Autodesk Fusion 360 part; units mm, degrees
(part 2 of 4)
sketch "Boceto28" plane through (0, 68, 0) normal (0, 1, 0) x (-1, 0, 0)
  line L0 (-4.7, -42.05) -> (43.7, -42.05)
  line L1 (43.7, -42.05) -> (43.7, -11.65)
  line L2 (43.7, -11.65) -> (-4.7, -11.65)
  line L3 (-4.7, -11.65) -> (-4.7, -42.05)
  line L4 (83, -73) -> (83, 19.3)
  line L5 (-44, -73) -> (83, -73)
  line L6 (-44, 19.3) -> (-44, -73)
  line L7 (83, 19.3) -> (-44, 19.3)
  line L8 (-33, -6.85) -> (72, -6.85)
  line L9 (72, -6.85) -> (72, -46.85)
  line L10 (72, -46.85) -> (-33, -46.85)
  line L11 (-33, -46.85) -> (-33, -6.85)
  line L12 (-33, -6.85) -> (72, -46.85) construction
  line L13 (72, -6.85) -> (-33, -46.85) construction
  point P0 (19.5, -26.85)
  point P1 (19.5, -26.85)
  dimension "d98" = 40
  dimension "d99" = 105
  constraint horizontal L8
  constraint perpendicular L8 L9
  constraint parallel L8 L10
  constraint parallel L9 L11
  constraint coincident L12 P1
  constraint coincident L13 P1
  constraint coincident P1 P0
  measures "d98" distance of L8.end L9.end
  measures "d99" distance of L9.end L10.end
extrude "Extruir27" add sketch "Boceto28" along normal blind 15 separate body contours L4 L5 L6 L7 makes body 3
sketch "Boceto29" plane through (0, 68, 0) normal (0, -1, 0) x (1, 0, 0)
  line L0 (33, -46.85) -> (-72, -46.85)
  line L1 (-72, -46.85) -> (-72, -6.85)
  line L2 (-72, -6.85) -> (33, -6.85)
  line L3 (33, -6.85) -> (33, -46.85)
  line L4 (44, 19.3) -> (-83, 19.3)
  line L5 (-83, 19.3) -> (-83, -73)
  line L6 (-83, -73) -> (44, -73)
  line L7 (44, -73) -> (44, 19.3)
  line L8 (33, -46.85) -> (33, -6.85)
  line L9 (-72, -46.85) -> (33, -46.85)
  line L10 (33, -6.85) -> (-72, -6.85)
  line L11 (-72, -6.85) -> (-72, -46.85)
  line L12 (-72, -6.85) -> (33, -6.85)
  line L13 (33, -6.85) -> (33, -46.85)
  line L14 (33, -46.85) -> (-72, -46.85)
  line L15 (-72, -46.85) -> (-72, -6.85)
  line L16 (30, -43.85) -> (-69, -43.85)
  line L17 (-69, -43.85) -> (-69, -9.85)
  line L18 (-69, -9.85) -> (30, -9.85)
  line L19 (30, -9.85) -> (30, -43.85)
  line L20 (-75, -49.85) -> (-75, -3.85)
  line L21 (-75, -3.85) -> (36, -3.85)
  line L22 (36, -3.85) -> (36, -49.85)
  line L23 (36, -49.85) -> (-75, -49.85)
  dimension "d102" = 3
  dimension "d103" = -3
  constraint horizontal L12
  constraint vertical L13
  constraint horizontal L14
  constraint vertical L15
  constraint coincident L0.start L3.end
  constraint coincident L1.end L2.start
extrude "Extruir28" add sketch "Boceto29" along normal blind 5 contours L0 L1 L2 L3 L8 L9 L10 L11 L12 L13 L14 L15 | L20 L21 L22 L23 bodies 3
sketch "Boceto30" plane through (0, 46, 0) normal (0, 1, 0) x (-1, 0, 0)
  line L0 (-41, -18.85) -> (-37, -18.85)
  line L1 (-37, -18.85) -> (-37, -22.85)
  line L2 (-37, -22.85) -> (-41, -22.85)
  line L3 (-41, -22.85) -> (-41, -30.85)
  line L4 (-41, -30.85) -> (-37, -30.85)
  line L5 (-37, -30.85) -> (-37, -34.85)
  line L6 (-37, -34.85) -> (-41, -34.85)
  line L7 (-41, -34.85) -> (-41, -70)
  line L8 (-41, -70) -> (80, -70)
  line L9 (80, -70) -> (80, -34.85)
  line L10 (80, -34.85) -> (76, -34.85)
  line L11 (76, -34.85) -> (76, -30.85)
  line L12 (76, -30.85) -> (80, -30.85)
  line L13 (80, -30.85) -> (80, -22.85)
  line L14 (80, -22.85) -> (76, -22.85)
  line L15 (76, -22.85) -> (76, -18.85)
  line L16 (76, -18.85) -> (80, -18.85)
  line L17 (80, -18.85) -> (80, 16.3)
  line L18 (80, 16.3) -> (-41, 16.3)
  line L19 (-41, 16.3) -> (-41, -18.85)
  line L20 (30, -11.35) -> (60, -11.35)
  line L21 (60, -11.35) -> (60, -42.35)
  line L22 (60, -42.35) -> (30, -42.35)
  line L23 (30, -42.35) -> (30, -43.35)
  line L24 (30, -43.35) -> (9, -43.35)
  line L25 (9, -43.35) -> (9, -10.35)
  line L26 (9, -10.35) -> (30, -10.35)
  line L27 (30, -10.35) -> (30, -11.35)
  line L28 (80, -70) -> (-41, 16.3)
  line L29 (80, 16.3) -> (-41, -70)
  line L30 (-41, 16.3) -> (-28.7879, 7.59)
  line L31 (-41, -70) -> (-28.7879, -61.29)
  line L32 (80, -70) -> (67.7879, -61.29) construction
  line L33 (80, 16.3) -> (67.7879, 7.59)
  circle A0 centre (67.7879, 7.59) radius 2.5
  circle A1 centre (67.7879, -61.29) radius 2.5
  circle A2 centre (-28.7879, -61.29) radius 2.5
  circle A3 centre (-28.7879, 7.59) radius 2.5
  dimension "d106" = 15
  dimension "d107" = 15
  dimension "d108" = 15
  dimension "d109" = 15
  dimension "d110" = 5
  dimension "d111" = 5
  dimension "d112" = 5
  dimension "d113" = 5
  constraint coincident L18.end L19.start
  constraint parallel L28 L30
  constraint coincident L7.end L8.start
  constraint parallel L29 L31
  constraint coincident L8.end L9.start
  constraint parallel L28 L32
  constraint coincident L17.end L18.start
  constraint parallel L29 L33
  constraint coincident L33.end A0.centre
  constraint coincident L32.end A1.centre
  constraint coincident L31.end A2.centre
  constraint coincident L30.end A3.centre
  measures "d106" distance of L18.end L30.end
  measures "d107" distance of L7.end L31.end
  measures "d108" distance of L8.end L32.end
  measures "d109" distance of L17.end L33.end
  measures "d110" diameter of A0
  measures "d111" diameter of A1
  measures "d112" diameter of A2
  measures "d113" diameter of A3
extrude "Extruir29" add sketch "Boceto30" along normal blind 21.99 contours L28 L30 A3 | L28 L30 A3 | L29 L33 A0 | L29 L33 A0 | L29 L31 A2 | L29 L31 A2 | L28 A1 | L28 A1 bodies 2
sketch "Boceto31" plane through (0, 68, 0) normal (0, -1, 0) x (1, 0, 0)
  line L0 (36, -49.85) -> (-75, -49.85)
  line L1 (-75, -49.85) -> (-75, -3.85)
  line L2 (-75, -3.85) -> (36, -3.85)
  line L3 (36, -3.85) -> (36, -49.85)
  line L4 (44, 19.3) -> (-83, 19.3)
  line L5 (-83, 19.3) -> (-83, -73)
  line L6 (-83, -73) -> (44, -73)
  line L7 (44, -73) -> (44, 19.3)
  circle A0 centre (-67.7879, -61.29) radius 2.5
  circle A1 centre (28.7879, -61.29) radius 2.5
  circle A2 centre (28.7879, 7.59) radius 2.5
  circle A3 centre (-67.7879, 7.59) radius 2.5
  circle A4 centre (28.7879, -61.29) radius 4
  circle A5 centre (-67.7879, -61.29) radius 4
  circle A6 centre (28.7879, -61.29) radius 2.5
  circle A7 centre (28.7879, 7.59) radius 2.5
  circle A8 centre (28.7879, 7.59) radius 2.5
  circle A9 centre (-67.7879, 7.59) radius 2.5
  circle A10 centre (28.7879, 7.59) radius 4
  circle A11 centre (-67.7879, 7.59) radius 4
  point P0 (28.7879, 7.59)
  dimension "d116" = 1.5
  dimension "d117" = 1.5
  dimension "d118" = 5
  dimension "d119" = 5
  dimension "d120" = 5
  dimension "d121" = 1.5
  dimension "d122" = 1.5
  constraint concentric A1 A6
  constraint coincident P0 A2.centre
  constraint concentric A2 A8
  constraint concentric A3 A9
  measures "d118" diameter of A6
  measures "d119" diameter of A8
  measures "d120" diameter of A9
extrude "Extruir30" add sketch "Boceto31" along normal blind 6 contours A4 | A5 | A10 | A11 bodies 3
sketch "Boceto32" plane through (0, 0, 19.3) normal (0, 0, 1) x (1, 0, 0)
  circle A0 centre (-18.2562, 20.244) radius 7.405
  line L0 (44, -4) -> (44, 64.2)
  line L1 (44, 64.2) -> (-83, 64.2)
  line L2 (-83, 64.2) -> (-83, -4)
  line L3 (-83, -4) -> (44, -4)
sketch "Boceto33" plane through (-83, 0, 0) normal (-1, 0, 0) x (0, 0, 1)
  line L0 (19.3, -4) -> (19.3, 64.2)
  line L1 (19.3, 64.2) -> (-73, 64.2)
  line L2 (-73, 64.2) -> (-73, -4)
  line L3 (-73, -4) -> (19.3, -4)
sketch "Boceto34" plane through (0, 0, 19.3) normal (0, 0, 1) x (1, 0, 0)
  line L0 (-34.8461, 5.5811) -> (-70.8461, 5.5811)
  line L1 (-70.8461, 5.5811) -> (-70.8461, 39.5811)
  line L2 (-70.8461, 39.5811) -> (-34.8461, 39.5811)
  line L3 (-34.8461, 39.5811) -> (-34.8461, 5.5811)
  line L4 (-34.8461, 5.5811) -> (-70.8461, 39.5811) construction
  line L5 (-70.8461, 5.5811) -> (-34.8461, 39.5811)
  line L6 (-52.8461, 5.5811) -> (-52.8461, 10.5811) construction
  line L7 (-70.3461, 33.5811) -> (-35.3461, 33.5811)
  line L8 (-35.3461, 33.5811) -> (-35.3461, 10.5811)
  line L9 (-35.3461, 10.5811) -> (-70.3461, 10.5811)
  line L10 (-70.3461, 10.5811) -> (-70.3461, 33.5811)
  line L11 (-70.3461, 33.5811) -> (-70.8461, 33.5811) construction
  line L12 (-70.8461, 5.5811) -> (-67.938, 8.3276)
  line L13 (-34.8461, 5.5811) -> (-37.7542, 8.3276)
  line L14 (-70.8461, 39.5811) -> (-67.938, 36.8346)
  line L15 (-34.8461, 39.5811) -> (-37.7542, 36.8346)
  circle A0 centre (-67.938, 8.3276) radius 1.5
  circle A1 centre (-37.7542, 8.3276) radius 1.5
  circle A2 centre (-67.938, 36.8346) radius 1.5
  circle A3 centre (-37.7542, 36.8346) radius 1.5
  line L16 (-70.3461, 33.5811) -> (-35.3461, 33.5811)
  line L17 (-35.3461, 33.5811) -> (-35.3461, 10.5811)
  line L18 (-35.3461, 10.5811) -> (-70.3461, 10.5811)
  line L19 (-70.3461, 10.5811) -> (-70.3461, 33.5811)
  point P0 (-52.8461, 22.5811)
  point P1 (-52.8461, 22.5811)
  dimension "d125" = 34
  dimension "d126" = 36
  dimension "d127" = 5
  dimension "d128" = 23
  dimension "d129" = 35
  dimension "d130" = 0.5
  dimension "d131" = 4
  dimension "d132" = 4
  dimension "d133" = 4
  dimension "d134" = 4
  dimension "d135" = 3
  dimension "d136" = 3
  dimension "d137" = 3
  dimension "d138" = 3
  constraint horizontal L0
  constraint perpendicular L0 L1
  constraint parallel L0 L2
  constraint parallel L1 L3
  constraint coincident L4 P1
  constraint coincident L5 P1
  constraint coincident P0 P1
  constraint midpoint L0 L6.start
  constraint perpendicular L0 L6
  constraint horizontal L7
  constraint vertical L8
  constraint horizontal L9
  constraint vertical L10
  constraint coincident L6.end L9
  constraint coincident L1 L11.end
  constraint perpendicular L1 L11
  constraint parallel L5 L12
  constraint parallel L4 L13
  constraint parallel L4 L14
  constraint parallel L5 L15
  constraint coincident L12.end A0.centre
  constraint coincident L13.end A1.centre
  constraint coincident L14.end A2.centre
  constraint coincident L15.end A3.centre
  constraint horizontal L16
  constraint vertical L17
  constraint horizontal L18
  constraint vertical L19
  measures "d125" distance of L0.end L1.end
  measures "d126" distance of L1.end L2.end
  measures "d127" distance of L6.start L6.end
  measures "d128" distance of L7.start L9.end
  measures "d129" distance of L7.start L7.end
  measures "d130" distance of L7.start L11.end
  measures "d131" distance of L0.end L12.end
  measures "d132" distance of L0.start L13.end
  measures "d133" distance of L1.end L14.end
  measures "d134" distance of L2.end L15.end
  measures "d135" diameter of A0
  measures "d136" diameter of A1
  measures "d137" diameter of A2
  measures "d138" diameter of A3
extrude "Extruir31" add sketch "Boceto34" against normal blind 9 contours L5 L12 A0 | L5 L12 A0 | L5 L15 A3 | L5 L15 A3 | A1 | A2 bodies 1
extrude "Extruir32" cut sketch "Boceto34" against normal blind 6 contours L5 L7 L9 L10 L16 L18 L19 | L5 L7 L8 L9 L16 L17 L18 bodies 1
sketch "Boceto35" plane through (0, 0, 0) normal (0, 1, 0) x (-1, 0, 0)
  line L0 (46.4591, -65.3063) -> (43.7876, -62.6347)
  line L1 (43.7876, -62.6347) -> (43.7876, -12.7779)
  line L2 (43.7876, -12.7779) -> (46.4591, -10.1063)
  line L3 (46.4591, -10.1063) -> (73.416, -10.1063)
  line L4 (73.416, -10.1063) -> (76.0876, -12.7779)
  line L5 (76.0876, -12.7779) -> (76.0876, -62.6347)
  line L6 (76.0876, -62.6347) -> (73.416, -65.3063)
  line L7 (73.416, -65.3063) -> (46.4591, -65.3063)
  line L8 (-41, 16.3) -> (-41, -70)
  line L9 (-41, -70) -> (80, -70)
  line L10 (80, -70) -> (80, 16.3)
  line L11 (80, 16.3) -> (-41, 16.3)
  line L12 (-38.4075, -60.7714) -> (-38.4075, -28.7305)
  line L13 (-38.4075, -28.7305) -> (19.6738, -28.7305)
  line L14 (19.6738, -28.7305) -> (19.6738, -60.7714)
  line L15 (19.6738, -60.7714) -> (-38.4075, -60.7714)
  line L16 (-21.368, 14.2774) -> (-27.5689, 14.2774)
  line L17 (-24.1184, -1.7226) -> (-24.1184, -0.7226)
  line L18 (-20.1184, -0.7226) -> (-18.6184, -0.7226)
  line L19 (-29.0184, -1.7226) -> (-29.0184, -0.7226)
  line L20 (-19.5184, -10.1726) -> (-22.0184, -10.1726)
  line L21 (-30.8184, 3.6774) -> (-30.8184, 5.0774)
  line L22 (-30.2184, -7.6726) -> (-30.2184, -10.1726)
  line L23 (-20.3184, 15.9774) -> (-21.368, 14.2774)
  line L24 (-32.7184, 12.4274) -> (-32.7184, 14.9274)
  line L25 (-22.1184, -1.7226) -> (-24.1184, -1.7226)
  line L26 (-30.8184, 5.0774) -> (-29.9184, 5.0774)
  line L27 (-29.6184, 9.9774) -> (-29.6184, 8.1774)
  line L28 (-29.6184, 8.1774) -> (-30.8184, 8.1774)
  line L29 (-33.1184, 15.9774) -> (-33.1184, -10.3226)
  line L30 (-30.2184, -10.1726) -> (-32.7184, -10.1726)
  line L31 (-27.5184, -1.7226) -> (-29.0184, -1.7226)
  line L32 (-22.0184, -10.1726) -> (-22.0184, -7.6726)
  line L33 (-29.9184, 5.0774) -> (-29.9184, 3.6774)
  line L34 (-30.8184, 8.1774) -> (-30.8184, 9.9774)
  line L35 (-30.8184, 9.9774) -> (-29.6184, 9.9774)
  line L36 (-18.8184, 3.7774) -> (-19.7184, 3.7774)
  line L37 (-18.6184, -0.7226) -> (-18.6184, -1.7226)
  line L38 (-19.7184, 3.7774) -> (-19.7184, 5.1774)
  line L39 (-22.1184, -0.7226) -> (-22.1184, -1.7226)
  line L40 (-19.7184, 5.1774) -> (-18.8184, 5.1774)
  line L41 (-18.8184, 9.7774) -> (-18.8184, 8.3774)
  line L42 (-18.8184, 8.3774) -> (-19.7184, 8.3774)
  line L43 (-19.7184, 8.3774) -> (-19.7184, 9.7774)
  line L44 (-18.8184, 5.1774) -> (-18.8184, 3.7774)
  line L45 (-19.7184, 9.7774) -> (-18.8184, 9.7774)
  line L46 (-15.8184, -10.3226) -> (-15.8184, 15.9774)
  line L47 (-33.1184, -10.3226) -> (-15.8184, -10.3226)
  line L48 (-30.2184, 14.9274) -> (-30.2184, 12.4274)
  line L49 (-30.2184, 12.4274) -> (-32.7184, 12.4274)
  line L50 (-27.5689, 14.2774) -> (-28.6184, 15.9774)
  line L51 (-29.4184, -7.6726) -> (-26.9184, -7.6726)
  line L52 (-32.7184, 14.9274) -> (-30.2184, 14.9274)
  line L53 (-28.6184, 15.9774) -> (-33.1184, 15.9774)
  line L54 (-16.2184, 14.9274) -> (-16.2184, 12.4274)
  line L55 (-22.0184, -7.6726) -> (-19.5184, -7.6726)
  line L56 (-19.5184, -7.6726) -> (-19.5184, -10.1726)
  line L57 (-18.7184, 12.4274) -> (-18.7184, 14.9274)
  line L58 (-24.1184, -0.7226) -> (-22.1184, -0.7226)
  line L59 (-22.1184, 0.6774) -> (-24.1184, 0.6774)
  line L60 (-24.1184, 1.6774) -> (-22.1184, 1.6774)
  line L61 (-15.8184, 15.9774) -> (-20.3184, 15.9774)
  line L62 (-32.7184, -7.6726) -> (-30.2184, -7.6726)
  line L63 (-26.9184, -7.6726) -> (-26.9184, -10.1726)
  line L64 (-18.7184, 14.9274) -> (-16.2184, 14.9274)
  line L65 (-16.2184, 12.4274) -> (-18.7184, 12.4274)
  line L66 (-32.7184, -10.1726) -> (-32.7184, -7.6726)
  line L67 (-27.5184, -0.7226) -> (-27.5184, -1.7226)
  line L68 (-29.0184, -0.7226) -> (-27.5184, -0.7226)
  line L69 (-24.1184, 0.6774) -> (-24.1184, 1.6774)
  line L70 (-29.9184, 3.6774) -> (-30.8184, 3.6774)
  line L71 (-29.4184, -10.1726) -> (-29.4184, -7.6726)
  line L72 (-26.9184, -10.1726) -> (-29.4184, -10.1726)
  line L73 (-18.6184, -1.7226) -> (-20.1184, -1.7226)
  line L74 (-22.1184, 1.6774) -> (-22.1184, 0.6774)
  line L75 (-20.1184, -1.7226) -> (-20.1184, -0.7226)
  line L76 (-23.4598, -8.7741) -> (-23.4598, -9.0434)
  line L77 (-23.1906, -9.0434) -> (-23.1906, -9.1588)
  spline S0 degree 3 poles (-23.0111, -8.4082) (-23.0132, -8.4184) (-23.0174, -8.4383) (-23.0264, -8.4666) (-23.038, -8.4923) (-23.0513, -8.5159) (-23.0675, -8.5367) (-23.0864, -8.5549) (-23.1077, -8.5709) (-23.1316, -8.584) (-23.1575, -8.5944) (-23.1849, -8.602) (-23.2138, -8.6065) (-23.2334, -8.6071) (-23.2435, -8.6075) knots 0 0 0 0 0.093348 0.18081 0.264145 0.343818 0.421385 0.498357 0.576984 0.657917 0.740639 0.825197 0.91066 1 1 1 1
  line L78 (-32.376, 1.6706) -> (-32.376, 1.2172)
  line L79 (-32.4914, 1.2415) -> (-32.4914, 1.8455)
  line L80 (-23.5752, -9.0434) -> (-23.5752, -8.7741)
  line L81 (-32.4914, 0.4031) -> (-32.2094, 0.4482)
  spline S1 degree 3 poles (-31.8408, 1.2717) (-31.8351, 1.2693) (-31.8237, 1.2643) (-31.8055, 1.2594) (-31.7866, 1.2563) (-31.7737, 1.2559) (-31.7673, 1.2557) knots 0 0 0 0 0.24526 0.491995 0.743436 1 1 1 1
  line L82 (-23.4598, -9.0434) -> (-23.1906, -9.0434)
  line L83 (-24.0111, -7.787) -> (-23.0111, -7.9939)
  spline S2 degree 3 poles (-31.4914, 1.4364) (-31.4918, 1.4223) (-31.4926, 1.3947) (-31.4996, 1.3545) (-31.5109, 1.3162) (-31.5264, 1.2802) (-31.546, 1.2474) (-31.5698, 1.2188) (-31.597, 1.1941) (-31.6278, 1.1748) (-31.6602, 1.1594) (-31.6938, 1.1486) (-31.7278, 1.1416) (-31.7508, 1.1407) (-31.7622, 1.1403) knots 0 0 0 0 0.09377 0.184231 0.27213 0.359606 0.445026 0.526727 0.607566 0.688585 0.76897 0.84681 0.923592 1 1 1 1
  spline S3 degree 3 poles (-25.5624, -8.5812) (-25.5645, -8.5915) (-25.5687, -8.6114) (-25.5777, -8.6397) (-25.5892, -8.6654) (-25.6026, -8.689) (-25.6187, -8.7098) (-25.6377, -8.728) (-25.659, -8.744) (-25.6829, -8.7571) (-25.7088, -8.7675) (-25.7362, -8.7751) (-25.7651, -8.7796) (-25.7847, -8.7802) (-25.7947, -8.7806) knots 0 0 0 0 0.093348 0.18081 0.264145 0.343818 0.421385 0.498357 0.576984 0.657917 0.740639 0.825197 0.91066 1 1 1 1
  spline S4 degree 3 poles (-32.4914, 1.8455) (-32.4772, 1.8421) (-32.4498, 1.8357) (-32.4109, 1.8232) (-32.3756, 1.8088) (-32.3433, 1.7924) (-32.3135, 1.7733) (-32.2846, 1.752) (-32.2566, 1.7277) (-32.2337, 1.7049) (-32.2146, 1.6839) (-32.1981, 1.6646) (-32.179, 1.6422) (-32.158, 1.6165) (-32.1348, 1.5874) (-32.1093, 1.5552) (-32.0817, 1.5195) (-32.0626, 1.4946) (-32.0527, 1.4817) knots 0 0 0 0 0.074725 0.144044 0.209069 0.269783 0.329265 0.390134 0.45341 0.518937 0.555488 0.598884 0.649104 0.705717 0.769214 0.839335 0.916353 1 1 1 1
  spline S5 degree 3 poles (-26.0373, -8.6271) (-26.042, -8.6383) (-26.051, -8.66) (-26.07, -8.6889) (-26.0921, -8.7134) (-26.1176, -8.7334) (-26.1458, -8.749) (-26.1766, -8.7596) (-26.2095, -8.7666) (-26.2322, -8.7673) (-26.2439, -8.7677) knots 0 0 0 0 0.135771 0.263552 0.384992 0.505027 0.624716 0.745551 0.869397 1 1 1 1
  line L84 (-23.4598, -9.428) -> (-23.5752, -9.428)
  line L85 (-32.2094, 0.8701) -> (-32.4914, 1.0225)
  spline S6 degree 3 poles (-31.6068, 1.4326) (-31.607, 1.4387) (-31.6073, 1.4506) (-31.6096, 1.4682) (-31.6131, 1.4853) (-31.6184, 1.5018) (-31.625, 1.5177) (-31.6333, 1.5329) (-31.6429, 1.5476) (-31.654, 1.5618) (-31.6667, 1.5752) (-31.6814, 1.5875) (-31.6979, 1.5989) (-31.7161, 1.6093) (-31.7361, 1.6185) (-31.7578, 1.6269) (-31.7814, 1.6343) (-31.7979, 1.6383) (-31.8063, 1.6403) knots 0 0 0 0 0.058001 0.11384 0.169165 0.223941 0.278457 0.333444 0.389076 0.445762 0.504761 0.564849 0.628439 0.695178 0.764689 0.838477 0.917221 1 1 1 1
  line L86 (-31.4914, 0.5967) -> (-31.4914, 0.459)
  spline S7 degree 3 poles (-25.7947, -8.7806) (-25.8082, -8.7801) (-25.8345, -8.7792) (-25.8727, -8.7721) (-25.9083, -8.7602) (-25.9359, -8.7464) (-25.9566, -8.7331) (-25.971, -8.7216) (-25.9845, -8.709) (-25.9969, -8.695) (-26.0086, -8.68) (-26.0192, -8.6635) (-26.0288, -8.6458) (-26.0345, -8.6334) (-26.0373, -8.6271) knots 0 0 0 0 0.13183 0.257674 0.379204 0.49925 0.559358 0.619481 0.679692 0.740425 0.802498 0.866422 0.932049 1 1 1 1
  spline S8 degree 3 poles (-23.486, -8.454) (-23.4907, -8.4652) (-23.4998, -8.4869) (-23.5187, -8.5158) (-23.5408, -8.5404) (-23.5663, -8.5603) (-23.5945, -8.5759) (-23.6253, -8.5866) (-23.6582, -8.5935) (-23.6809, -8.5943) (-23.6926, -8.5947) knots 0 0 0 0 0.135771 0.263552 0.384992 0.505027 0.624716 0.745551 0.869397 1 1 1 1
  spline S9 degree 3 poles (-31.7891, 1.7557) (-31.7778, 1.754) (-31.7558, 1.7506) (-31.7239, 1.743) (-31.6938, 1.7332) (-31.6656, 1.7212) (-31.6391, 1.7071) (-31.6144, 1.6909) (-31.5916, 1.6723) (-31.5709, 1.6517) (-31.5522, 1.6295) (-31.536, 1.6058) (-31.5219, 1.5809) (-31.5111, 1.5544) (-31.502, 1.5269) (-31.496, 1.4978) (-31.492, 1.4676) (-31.4916, 1.4469) (-31.4914, 1.4364) knots 0 0 0 0 0.070842 0.138839 0.204079 0.267816 0.329596 0.390853 0.451462 0.512345 0.572577 0.632109 0.691133 0.750229 0.81008 0.871347 0.93465 1 1 1 1
  spline S10 degree 3 poles (-32.1759, 1.4674) (-32.1816, 1.4748) (-32.1928, 1.4891) (-32.2092, 1.5097) (-32.2248, 1.529) (-32.2396, 1.5468) (-32.2536, 1.563) (-32.2669, 1.5779) (-32.2792, 1.5913) (-32.2945, 1.6068) (-32.3127, 1.6242) (-32.3343, 1.6423) (-32.355, 1.6579) (-32.3692, 1.6665) (-32.376, 1.6706) knots 0 0 0 0 0.097505 0.189443 0.27582 0.356648 0.431407 0.50065 0.564397 0.622172 0.728871 0.826509 0.916873 1 1 1 1
  spline S11 degree 3 poles (-31.8247, 2.205) (-31.825, 2.1959) (-31.8254, 2.1781) (-31.8291, 2.1519) (-31.835, 2.1269) (-31.8438, 2.1032) (-31.8546, 2.0806) (-31.8679, 2.0592) (-31.8839, 2.0392) (-31.9018, 2.0203) (-31.922, 2.0034) (-31.9439, 1.9884) (-31.9678, 1.976) (-31.9931, 1.9658) (-32.0201, 1.9577) (-32.0489, 1.9522) (-32.0792, 1.9487) (-32.1, 1.9483) (-32.1106, 1.948) knots 0 0 0 0 0.063114 0.12396 0.183107 0.241334 0.29898 0.356871 0.415955 0.47629 0.537492 0.598572 0.660371 0.723392 0.788226 0.855783 0.926232 1 1 1 1
  spline S12 degree 3 poles (-31.9421, 1.3473) (-31.9337, 1.339) (-31.9175, 1.3232) (-31.8918, 1.3026) (-31.8668, 1.2849) (-31.8492, 1.276) (-31.8408, 1.2717) knots 0 0 0 0 0.277808 0.535709 0.776314 1 1 1 1
  spline S13 degree 3 poles (-31.7673, 1.2557) (-31.7618, 1.2559) (-31.7509, 1.2562) (-31.735, 1.2586) (-31.7198, 1.2626) (-31.7052, 1.2683) (-31.6912, 1.2755) (-31.6778, 1.2842) (-31.6652, 1.2947) (-31.6532, 1.3067) (-31.6423, 1.3197) (-31.6328, 1.3337) (-31.6248, 1.3484) (-31.6181, 1.3638) (-31.6131, 1.38) (-31.6095, 1.3969) (-31.6073, 1.4145) (-31.607, 1.4265) (-31.6068, 1.4326) knots 0 0 0 0 0.061831 0.122011 0.181198 0.23938 0.298663 0.357989 0.419511 0.483417 0.548121 0.610998 0.67369 0.736783 0.799907 0.864607 0.931398 1 1 1 1
  spline S14 degree 3 poles (-32.5042, 2.2814) (-32.504, 2.2913) (-32.5035, 2.3107) (-32.4991, 2.3391) (-32.4922, 2.3664) (-32.482, 2.3923) (-32.4694, 2.417) (-32.4536, 2.4402) (-32.4352, 2.4625) (-32.4141, 2.4832) (-32.3902, 2.502) (-32.364, 2.5186) (-32.3353, 2.5327) (-32.304, 2.5437) (-32.2705, 2.5526) (-32.2347, 2.5589) (-32.1964, 2.5628) (-32.17, 2.5632) (-32.1565, 2.5634) knots 0 0 0 0 0.058939 0.115647 0.171125 0.22616 0.28078 0.336385 0.393175 0.452247 0.512572 0.573713 0.637048 0.702606 0.770921 0.843255 0.919213 1 1 1 1
  spline S15 degree 3 poles (-31.8474, 2.5109) (-31.8373, 2.5075) (-31.8177, 2.5008) (-31.7889, 2.49) (-31.7617, 2.4784) (-31.7358, 2.4661) (-31.7112, 2.4533) (-31.6878, 2.4402) (-31.666, 2.4261) (-31.639, 2.407) (-31.6086, 2.3822) (-31.5766, 2.351) (-31.5497, 2.319) (-31.5281, 2.2855) (-31.5116, 2.2505) (-31.5, 2.2136) (-31.4927, 2.1745) (-31.4919, 2.1476) (-31.4914, 2.1339) knots 0 0 0 0 0.057149 0.112173 0.165396 0.216763 0.266676 0.314719 0.36135 0.406796 0.492759 0.572434 0.64733 0.717927 0.786365 0.85547 0.926079 1 1 1 1
  line L87 (-26.2675, -8.8703) -> (-26.1521, -8.8959)
  spline S16 degree 3 poles (-31.4914, 2.1339) (-31.4916, 2.1257) (-31.4919, 2.1096) (-31.4951, 2.0861) (-31.4998, 2.0636) (-31.5069, 2.0424) (-31.5157, 2.0222) (-31.5265, 2.0033) (-31.5395, 1.9855) (-31.5542, 1.9689) (-31.571, 1.9539) (-31.5893, 1.9403) (-31.6094, 1.9287) (-31.6314, 1.919) (-31.6549, 1.9107) (-31.6801, 1.9041) (-31.7069, 1.8993) (-31.7255, 1.8976) (-31.735, 1.8967) knots 0 0 0 0 0.064924 0.127135 0.18703 0.245903 0.303523 0.360697 0.418085 0.476731 0.535729 0.595328 0.656298 0.719326 0.784711 0.852895 0.924692 1 1 1 1
  spline S17 degree 3 poles (-31.7478, 2.0103) (-31.7418, 2.0112) (-31.7302, 2.0128) (-31.7135, 2.0165) (-31.698, 2.0207) (-31.6839, 2.0264) (-31.6708, 2.0321) (-31.6593, 2.0393) (-31.649, 2.0471) (-31.6371, 2.0585) (-31.6248, 2.0746) (-31.6146, 2.0963) (-31.6077, 2.1198) (-31.6071, 2.1363) (-31.6068, 2.1447) knots 0 0 0 0 0.084332 0.162968 0.237114 0.306581 0.372865 0.434796 0.494241 0.551869 0.663534 0.772448 0.882971 1 1 1 1
  line L88 (-23.8444, -9.1588) -> (-23.8444, -9.0434)
  line L89 (-23.5752, -9.1588) -> (-23.8444, -9.1588)
  line L90 (-23.8444, -9.0434) -> (-23.5752, -9.0434)
  line L91 (-23.5752, -9.428) -> (-23.5752, -9.1588)
  spline S18 degree 3 poles (-32.1106, 1.948) (-32.1244, 1.9483) (-32.1518, 1.9488) (-32.1919, 1.9543) (-32.2305, 1.9626) (-32.2677, 1.9742) (-32.3032, 1.9896) (-32.3374, 2.008) (-32.3701, 2.0299) (-32.3903, 2.047) (-32.4005, 2.0556) knots 0 0 0 0 0.131174 0.258883 0.383336 0.505499 0.627474 0.749873 0.873513 1 1 1 1
  line L92 (-23.5752, -8.7741) -> (-23.4598, -8.7741)
  line L93 (-25.5624, -8.167) -> (-25.5624, -8.5812)
  line L94 (-26.5624, -8.4304) -> (-26.5624, -7.96)
  line L95 (-23.1906, -9.1588) -> (-23.4598, -9.1588)
  line L96 (-23.4598, -9.1588) -> (-23.4598, -9.428)
  line L97 (-23.0111, -7.9939) -> (-23.0111, -8.4082)
  line L98 (-32.4914, 1.0225) -> (-32.4914, 1.1517)
  line L99 (-31.4914, 0.459) -> (-32.4914, 0.2866)
  line L100 (-26.1521, -8.8959) -> (-26.1521, -9.2806)
  line L101 (-32.4914, 0.2866) -> (-32.4914, 0.4031)
  line L102 (-32.376, 1.2172) -> (-32.4914, 1.2415)
  spline S19 degree 3 poles (-23.2435, -8.6075) (-23.2569, -8.607) (-23.2832, -8.6061) (-23.3214, -8.599) (-23.357, -8.5871) (-23.3846, -8.5733) (-23.4053, -8.5601) (-23.4197, -8.5486) (-23.4332, -8.5359) (-23.4456, -8.522) (-23.4573, -8.5069) (-23.4679, -8.4905) (-23.4776, -8.4728) (-23.4832, -8.4603) (-23.486, -8.454) knots 0 0 0 0 0.13183 0.257674 0.379204 0.49925 0.559358 0.619481 0.679692 0.740425 0.802498 0.866422 0.932049 1 1 1 1
  line L103 (-24.0111, -8.2573) -> (-24.0111, -7.787)
  spline S20 degree 3 poles (-32.0527, 1.4817) (-32.0467, 1.4738) (-32.0352, 1.4585) (-32.0181, 1.437) (-32.0026, 1.4171) (-31.9881, 1.3995) (-31.9749, 1.3836) (-31.963, 1.3697) (-31.9523, 1.3577) (-31.9454, 1.3506) (-31.9421, 1.3473) knots 0 0 0 0 0.17071 0.328805 0.473784 0.604575 0.722989 0.829042 0.920272 1 1 1 1
  spline S21 degree 3 poles (-31.6068, 2.1447) (-31.6073, 2.1539) (-31.6083, 2.1727) (-31.6169, 2.2008) (-31.6307, 2.2286) (-31.6493, 2.2564) (-31.6732, 2.2833) (-31.7027, 2.3081) (-31.7369, 2.3313) (-31.7756, 2.3512) (-31.8153, 2.3692) (-31.8538, 2.3846) (-31.89, 2.3972) (-31.9137, 2.4031) (-31.9251, 2.406) knots 0 0 0 0 0.062676 0.128115 0.197983 0.274152 0.355774 0.442669 0.536146 0.637202 0.738709 0.833348 0.919908 1 1 1 1
  line L104 (-32.4914, 1.1517) -> (-31.4914, 0.5967)
  spline S22 degree 3 poles (-31.9251, 2.406) (-31.9171, 2.3977) (-31.9015, 2.3816) (-31.8814, 2.3559) (-31.8636, 2.3308) (-31.8497, 2.3054) (-31.8384, 2.2803) (-31.8306, 2.2551) (-31.8257, 2.2301) (-31.8251, 2.2133) (-31.8247, 2.205) knots 0 0 0 0 0.150106 0.291203 0.424345 0.54968 0.66843 0.78229 0.891952 1 1 1 1
  line L105 (-32.2094, 0.4482) -> (-32.2094, 0.8701)
  spline S23 degree 3 poles (-32.4005, 2.0556) (-32.4087, 2.0634) (-32.4249, 2.0787) (-32.4462, 2.1039) (-32.4641, 2.1305) (-32.4789, 2.1582) (-32.4901, 2.1873) (-32.4984, 2.2175) (-32.5033, 2.249) (-32.5039, 2.2705) (-32.5042, 2.2814) knots 0 0 0 0 0.132591 0.260636 0.385015 0.506986 0.627697 0.749187 0.872499 1 1 1 1
  spline S24 degree 3 poles (-23.6926, -8.5947) (-23.7063, -8.5942) (-23.7338, -8.5932) (-23.7744, -8.5837) (-23.8143, -8.5696) (-23.8523, -8.5492) (-23.888, -8.5247) (-23.9199, -8.4959) (-23.9475, -8.4633) (-23.9702, -8.4271) (-23.9886, -8.388) (-24.0016, -8.3464) (-24.0097, -8.3026) (-24.0106, -8.2726) (-24.0111, -8.2573) knots 0 0 0 0 0.079881 0.159871 0.241278 0.325617 0.41027 0.493115 0.575047 0.657876 0.741532 0.825508 0.91122 1 1 1 1
  line L106 (-26.1521, -9.2806) -> (-26.2675, -9.2549)
  spline S25 degree 3 poles (-31.7622, 1.1403) (-31.7706, 1.1406) (-31.7874, 1.1411) (-31.8124, 1.1443) (-31.8372, 1.15) (-31.8616, 1.1579) (-31.8859, 1.1678) (-31.9099, 1.18) (-31.9336, 1.1945) (-31.9488, 1.2056) (-31.9566, 1.2112) knots 0 0 0 0 0.119036 0.238906 0.358896 0.480728 0.60402 0.732065 0.863551 1 1 1 1
  line L107 (-31.8063, 1.6403) -> (-31.7891, 1.7557)
  spline S26 degree 3 poles (-31.9566, 1.2112) (-31.959, 1.2133) (-31.9644, 1.2177) (-31.9726, 1.2252) (-31.9817, 1.2338) (-31.9916, 1.2439) (-32.0022, 1.2555) (-32.0139, 1.2681) (-32.0262, 1.2822) (-32.0396, 1.2975) (-32.0537, 1.3142) (-32.0687, 1.3322) (-32.0845, 1.3514) (-32.1011, 1.3721) (-32.1187, 1.394) (-32.137, 1.4174) (-32.1562, 1.442) (-32.1692, 1.4588) (-32.1759, 1.4674) knots 0 0 0 0 0.028628 0.061383 0.098297 0.140656 0.186818 0.237606 0.293065 0.353601 0.417996 0.487479 0.561215 0.639668 0.723216 0.810657 0.903196 1 1 1 1
  spline S27 degree 3 poles (-32.1565, 2.5634) (-32.144, 2.5632) (-32.1188, 2.5629) (-32.0809, 2.5605) (-32.0427, 2.5562) (-32.0042, 2.5507) (-31.9654, 2.5431) (-31.9262, 2.5342) (-31.8868, 2.5233) (-31.8606, 2.5151) (-31.8474, 2.5109) knots 0 0 0 0 0.119009 0.239505 0.361764 0.48522 0.610255 0.738208 0.868176 1 1 1 1
  line L108 (-31.735, 1.8967) -> (-31.7478, 2.0103)
  line L109 (-26.5624, -7.96) -> (-25.5624, -8.167)
  spline S28 degree 3 poles (-26.2439, -8.7677) (-26.2576, -8.7672) (-26.2851, -8.7662) (-26.3256, -8.7568) (-26.3655, -8.7427) (-26.4036, -8.7223) (-26.4393, -8.6978) (-26.4712, -8.6689) (-26.4988, -8.6364) (-26.5215, -8.6002) (-26.5399, -8.5611) (-26.5529, -8.5195) (-26.5609, -8.4756) (-26.5619, -8.4456) (-26.5624, -8.4304) knots 0 0 0 0 0.079881 0.159871 0.241278 0.325617 0.41027 0.493115 0.575047 0.657876 0.741532 0.825508 0.91122 1 1 1 1
  line L110 (-26.2675, -9.2549) -> (-26.2675, -8.8703)
  spline S29 degree 3 poles (-31.4914, 3.7158) (-31.4916, 3.7061) (-31.4921, 3.687) (-31.4956, 3.6592) (-31.5011, 3.6327) (-31.5092, 3.6076) (-31.5196, 3.584) (-31.5321, 3.5617) (-31.547, 3.541) (-31.5642, 3.5219) (-31.5829, 3.5045) (-31.603, 3.4895) (-31.624, 3.4767) (-31.6461, 3.4663) (-31.6693, 3.4579) (-31.6936, 3.4522) (-31.7189, 3.4487) (-31.7361, 3.4483) (-31.7448, 3.448) knots 0 0 0 0 0.070883 0.138331 0.203787 0.26699 0.329542 0.390794 0.452316 0.514838 0.576969 0.637605 0.696589 0.75561 0.814835 0.875193 0.936387 1 1 1 1
  spline S30 degree 3 poles (-32.11, 3.2162) (-32.1032, 3.2235) (-32.0897, 3.238) (-32.0662, 3.2564) (-32.0408, 3.2721) (-32.0133, 3.2851) (-31.9835, 3.2947) (-31.9517, 3.3021) (-31.9177, 3.3062) (-31.8943, 3.3067) (-31.8822, 3.307) knots 0 0 0 0 0.117536 0.23472 0.352011 0.470977 0.594371 0.722632 0.857423 1 1 1 1
  spline S31 degree 3 poles (-31.9121, 3.8148) (-31.9128, 3.8091) (-31.9142, 3.7978) (-31.9144, 3.7865) (-31.9145, 3.781) knots 0 0 0 0 0.510074 1 1 1 1
  spline S32 degree 3 poles (-32.0299, 3.7966) (-32.0301, 3.7986) (-32.0306, 3.8036) (-32.0333, 3.8121) (-32.0373, 3.8232) (-32.0408, 3.8313) (-32.0427, 3.8358) knots 0 0 0 0 0.146231 0.361927 0.644689 1 1 1 1
  line L111 (-32.1898, -6.2757) -> (-32.1898, -6.8526)
  line L112 (-31.8436, -5.718) -> (-31.709, -5.7564)
  line L113 (-31.709, -5.8911) -> (-31.4359, -5.9436)
  spline S33 degree 3 poles (-32.3888, 3.1149) (-32.3886, 3.1093) (-32.3882, 3.0981) (-32.3854, 3.0815) (-32.3804, 3.0652) (-32.3739, 3.0491) (-32.3652, 3.0334) (-32.3544, 3.0181) (-32.342, 3.003) (-32.3326, 2.9936) (-32.3277, 2.9887) knots 0 0 0 0 0.116883 0.23243 0.349774 0.469977 0.593693 0.722391 0.857554 1 1 1 1
  line L114 (-32.6591, -6.0563) -> (-32.8094, -6.026)
  spline S34 degree 3 poles (-32.5042, 3.1227) (-32.504, 3.1309) (-32.5037, 3.1469) (-32.5006, 3.1704) (-32.4956, 3.1927) (-32.4886, 3.2139) (-32.4795, 3.2338) (-32.4687, 3.2528) (-32.4556, 3.2705) (-32.4405, 3.2869) (-32.4237, 3.3018) (-32.4054, 3.3155) (-32.3851, 3.3268) (-32.3636, 3.337) (-32.34, 3.3449) (-32.3151, 3.3513) (-32.2884, 3.356) (-32.2701, 3.3575) (-32.2606, 3.3583) knots 0 0 0 0 0.064627 0.12706 0.187282 0.245862 0.30342 0.360798 0.418703 0.47752 0.537123 0.596934 0.657857 0.720848 0.785792 0.854086 0.925004 1 1 1 1
  spline S35 degree 3 poles (-31.4914, 2.9793) (-31.4917, 2.9696) (-31.4922, 2.9505) (-31.4965, 2.9226) (-31.5036, 2.896) (-31.5139, 2.8707) (-31.5264, 2.8465) (-31.5423, 2.8237) (-31.5611, 2.8023) (-31.5822, 2.7819) (-31.6063, 2.7638) (-31.6326, 2.7476) (-31.6615, 2.7342) (-31.6927, 2.7235) (-31.7261, 2.7148) (-31.7619, 2.7087) (-31.8, 2.7051) (-31.8263, 2.7047) (-31.8398, 2.7044) knots 0 0 0 0 0.058314 0.114386 0.169734 0.223814 0.278257 0.333412 0.39036 0.449174 0.50967 0.571329 0.634764 0.700697 0.769579 0.842158 0.918822 1 1 1 1
  line L115 (-31.709, -6.2564) -> (-31.8436, -6.218)
  line L116 (-31.8436, -6.218) -> (-31.8436, -6.0257)
  spline S36 degree 3 poles (-31.8822, 3.307) (-31.8685, 3.3067) (-31.8414, 3.3062) (-31.8015, 3.3009) (-31.7631, 3.2929) (-31.7263, 3.2811) (-31.6908, 3.2662) (-31.6569, 3.2482) (-31.6244, 3.2267) (-31.6044, 3.2099) (-31.5944, 3.2014) knots 0 0 0 0 0.13167 0.259135 0.383905 0.506516 0.628457 0.750748 0.874216 1 1 1 1
  spline S37 degree 3 poles (-32.1593, 2.7571) (-32.1743, 2.7624) (-32.2035, 2.7728) (-32.2454, 2.7904) (-32.2841, 2.8098) (-32.3201, 2.8299) (-32.3526, 2.8523) (-32.3824, 2.8754) (-32.4093, 2.9) (-32.4249, 2.9179) (-32.4325, 2.9268) knots 0 0 0 0 0.146713 0.285622 0.418201 0.544915 0.665352 0.781008 0.892429 1 1 1 1
  line L117 (-31.7729, 3.9096) -> (-31.7508, 4.0249)
  line L118 (-32.2222, 4.1531) -> (-32.2094, 4.0378)
  spline S38 degree 3 poles (-31.7448, 3.448) (-31.7512, 3.4481) (-31.7638, 3.4483) (-31.7825, 3.4504) (-31.8004, 3.4538) (-31.8178, 3.4584) (-31.8346, 3.4644) (-31.8507, 3.4716) (-31.8662, 3.4803) (-31.8861, 3.4938) (-31.9097, 3.5139) (-31.9353, 3.5429) (-31.9582, 3.5768) (-31.9709, 3.6019) (-31.9774, 3.6149) knots 0 0 0 0 0.063286 0.124263 0.184614 0.243272 0.302045 0.359849 0.417961 0.476807 0.596948 0.722967 0.856745 1 1 1 1
  line L119 (-31.8436, -6.0257) -> (-32.4746, -5.8911)
  line L120 (-32.0427, 3.8358) -> (-31.9121, 3.8148)
  spline S39 degree 3 poles (-31.7538, 3.5634) (-31.7487, 3.5636) (-31.7387, 3.5639) (-31.724, 3.5662) (-31.71, 3.5697) (-31.6965, 3.5748) (-31.6837, 3.5815) (-31.6715, 3.5894) (-31.66, 3.5991) (-31.649, 3.6097) (-31.6391, 3.6217) (-31.6304, 3.6343) (-31.6232, 3.6477) (-31.6171, 3.6615) (-31.6126, 3.6762) (-31.6091, 3.6915) (-31.6071, 3.7074) (-31.6069, 3.7182) (-31.6068, 3.7237) knots 0 0 0 0 0.062918 0.123951 0.183704 0.242051 0.301581 0.361887 0.422964 0.486687 0.551256 0.614315 0.676468 0.738671 0.801947 0.86633 0.932163 1 1 1 1
  line L121 (-32.2606, 3.3583) -> (-32.2478, 3.2433)
  line L122 (-32.3628, -6.8141) -> (-32.3628, -6.2372)
  spline S40 degree 3 poles (-32.4746, -5.8911) (-32.4841, -5.8893) (-32.5021, -5.886) (-32.5277, -5.8819) (-32.5503, -5.8782) (-32.5699, -5.8753) (-32.5864, -5.8728) (-32.5998, -5.8709) (-32.6103, -5.87) (-32.6163, -5.8698) (-32.6189, -5.8697) knots 0 0 0 0 0.198784 0.376221 0.532667 0.670161 0.782601 0.87611 0.948465 1 1 1 1
  spline S41 degree 3 poles (-32.6189, -5.8697) (-32.6243, -5.8699) (-32.6345, -5.8704) (-32.6489, -5.8737) (-32.6614, -5.8791) (-32.6719, -5.8871) (-32.6803, -5.8981) (-32.686, -5.912) (-32.6891, -5.929) (-32.6895, -5.9412) (-32.6898, -5.9478) knots 0 0 0 0 0.133915 0.253294 0.361774 0.467629 0.576952 0.697757 0.836473 1 1 1 1
  line L123 (-32.8051, -5.1603) -> (-32.6068, -5.2008)
  spline S42 degree 3 poles (-32.6068, -5.2008) (-32.6241, -5.1855) (-32.6576, -5.1558) (-32.7016, -5.1082) (-32.7395, -5.0608) (-32.7703, -5.013) (-32.7945, -4.9648) (-32.8116, -4.9164) (-32.8225, -4.8676) (-32.8238, -4.8349) (-32.8244, -4.8186) knots 0 0 0 0 0.152822 0.295762 0.428272 0.553392 0.670988 0.784111 0.892453 1 1 1 1
  spline S43 degree 3 poles (-32.5042, 3.8406) (-32.504, 3.8517) (-32.5036, 3.8733) (-32.4999, 3.905) (-32.4939, 3.935) (-32.4855, 3.9634) (-32.4747, 3.9901) (-32.4613, 4.0152) (-32.4458, 4.0387) (-32.4277, 4.0603) (-32.4076, 4.0799) (-32.3859, 4.0974) (-32.3626, 4.1127) (-32.3376, 4.1256) (-32.311, 4.136) (-32.2829, 4.1443) (-32.2531, 4.1501) (-32.2326, 4.1521) (-32.2222, 4.1531) knots 0 0 0 0 0.07053 0.138459 0.203385 0.266232 0.32755 0.387555 0.447622 0.507676 0.567486 0.626727 0.685967 0.745576 0.80618 0.868496 0.932919 1 1 1 1
  line L124 (-31.709, -5.7564) -> (-31.709, -5.8911)
  spline S44 degree 3 poles (-32.8244, -4.8186) (-32.8241, -4.8089) (-32.8237, -4.7899) (-32.8203, -4.7621) (-32.8149, -4.7356) (-32.8076, -4.7106) (-32.7974, -4.6872) (-32.7853, -4.6652) (-32.7713, -4.6443) (-32.7547, -4.6255) (-32.7367, -4.6085) (-32.7178, -4.5933) (-32.6978, -4.5806) (-32.6768, -4.5701) (-32.6547, -4.5619) (-32.6317, -4.5562) (-32.6077, -4.5528) (-32.5914, -4.5524) (-32.5831, -4.5521) knots 0 0 0 0 0.072499 0.141692 0.208769 0.273502 0.336062 0.398225 0.460571 0.523024 0.584826 0.64489 0.70331 0.761755 0.819879 0.878381 0.937945 1 1 1 1
  spline S45 degree 3 poles (-32.5831, -4.5521) (-32.5768, -4.5522) (-32.5631, -4.5525) (-32.5411, -4.5545) (-32.516, -4.5576) (-32.4876, -4.5613) (-32.4564, -4.5671) (-32.4218, -4.5731) (-32.3843, -4.5812) (-32.3581, -4.5868) (-32.3445, -4.5897) knots 0 0 0 0 0.078305 0.169301 0.274392 0.392282 0.523404 0.668633 0.827246 1 1 1 1
  spline S46 degree 3 poles (-32.1735, 3.4993) (-32.1845, 3.4996) (-32.2062, 3.5003) (-32.2382, 3.5049) (-32.2691, 3.513) (-32.2989, 3.5241) (-32.3276, 3.5381) (-32.355, 3.5556) (-32.3813, 3.5761) (-32.4063, 3.5995) (-32.4291, 3.6251) (-32.4493, 3.6522) (-32.4662, 3.6806) (-32.4801, 3.7102) (-32.491, 3.7411) (-32.4985, 3.7732) (-32.5033, 3.8065) (-32.5039, 3.8291) (-32.5042, 3.8406) knots 0 0 0 0 0.062371 0.123398 0.183837 0.243813 0.303951 0.365075 0.428142 0.493716 0.559362 0.62318 0.685525 0.74721 0.808842 0.87131 0.934593 1 1 1 1
  spline S47 degree 3 poles (-32.7691, -5.7384) (-32.7618, -5.7312) (-32.7472, -5.7169) (-32.7198, -5.702) (-32.6887, -5.6931) (-32.6667, -5.6921) (-32.6552, -5.6915) knots 0 0 0 0 0.241533 0.480086 0.728963 1 1 1 1
  line L125 (-31.8436, -5.8526) -> (-31.8436, -5.718)
  spline S48 degree 3 poles (-32.1709, 3.0606) (-32.1707, 3.0678) (-32.1703, 3.0819) (-32.1674, 3.1029) (-32.1626, 3.1233) (-32.156, 3.1432) (-32.1473, 3.1624) (-32.1368, 3.1811) (-32.1244, 3.1992) (-32.1148, 3.2105) (-32.11, 3.2162) knots 0 0 0 0 0.125493 0.248433 0.371194 0.49234 0.615576 0.740405 0.868442 1 1 1 1
  spline S49 degree 3 poles (-32.2478, 3.2433) (-32.254, 3.2423) (-32.2659, 3.2403) (-32.283, 3.2366) (-32.2986, 3.232) (-32.3129, 3.2266) (-32.3258, 3.2203) (-32.3375, 3.2137) (-32.3476, 3.2059) (-32.3593, 3.1951) (-32.371, 3.1798) (-32.3816, 3.1598) (-32.3877, 3.1378) (-32.3885, 3.1226) (-32.3888, 3.1149) knots 0 0 0 0 0.088726 0.171482 0.248748 0.320922 0.388489 0.452369 0.51204 0.569183 0.67885 0.783819 0.890321 1 1 1 1
  spline S50 degree 3 poles (-31.5944, 3.2014) (-31.5862, 3.1938) (-31.5701, 3.1789) (-31.5491, 3.1542) (-31.5313, 3.1282) (-31.5168, 3.1009) (-31.5052, 3.0724) (-31.4973, 3.0425) (-31.4923, 3.0113) (-31.4917, 2.99) (-31.4914, 2.9793) knots 0 0 0 0 0.132236 0.260368 0.384091 0.505313 0.626545 0.748013 0.872282 1 1 1 1
  spline S51 degree 3 poles (-32.2094, 4.0378) (-32.2171, 4.0365) (-32.2322, 4.0342) (-32.2537, 4.0288) (-32.2736, 4.0227) (-32.2918, 4.0154) (-32.3082, 4.0069) (-32.3229, 3.9975) (-32.3361, 3.9871) (-32.3473, 3.9753) (-32.3572, 3.9626) (-32.3657, 3.949) (-32.3729, 3.9345) (-32.3787, 3.9189) (-32.3834, 3.9025) (-32.3864, 3.8851) (-32.3886, 3.8668) (-32.3888, 3.8543) (-32.3888, 3.8479) knots 0 0 0 0 0.080927 0.15663 0.227951 0.295487 0.358216 0.417906 0.475134 0.530562 0.585433 0.639798 0.695756 0.752324 0.810213 0.871029 0.933968 1 1 1 1
  spline S52 degree 3 poles (-31.6068, 3.7237) (-31.6074, 3.7344) (-31.6085, 3.7556) (-31.6167, 3.7866) (-31.6307, 3.8156) (-31.6463, 3.838) (-31.6613, 3.8547) (-31.674, 3.8661) (-31.6876, 3.8764) (-31.7025, 3.8854) (-31.7185, 3.8932) (-31.7355, 3.9001) (-31.7538, 3.9054) (-31.7664, 3.9082) (-31.7729, 3.9096) knots 0 0 0 0 0.118513 0.234491 0.351331 0.472716 0.535406 0.598096 0.660816 0.724724 0.789733 0.857285 0.927326 1 1 1 1
  spline S53 degree 3 poles (-31.7508, 4.0249) (-31.7408, 4.0223) (-31.721, 4.0172) (-31.6926, 4.0074) (-31.6659, 3.9959) (-31.641, 3.9827) (-31.6178, 3.9677) (-31.5963, 3.9511) (-31.5766, 3.9329) (-31.5589, 3.9129) (-31.543, 3.8916) (-31.5292, 3.8694) (-31.5175, 3.8462) (-31.508, 3.822) (-31.5007, 3.7968) (-31.4952, 3.7707) (-31.4919, 3.7436) (-31.4916, 3.7252) (-31.4914, 3.7158) knots 0 0 0 0 0.071024 0.139634 0.205304 0.269463 0.332554 0.393764 0.454846 0.515989 0.576371 0.636066 0.694893 0.753756 0.813735 0.874378 0.936016 1 1 1 1
  spline S54 degree 3 poles (-31.8201, 4.2044) (-31.8338, 4.2046) (-31.8612, 4.2048) (-31.9021, 4.2077) (-31.9431, 4.2114) (-31.9838, 4.2177) (-32.0246, 4.2249) (-32.0651, 4.2343) (-32.1056, 4.245) (-32.1323, 4.2535) (-32.1457, 4.2577) knots 0 0 0 0 0.123997 0.247616 0.371576 0.496272 0.621059 0.746345 0.872794 1 1 1 1
  spline S55 degree 3 poles (-32.1457, 4.2577) (-32.1611, 4.263) (-32.1914, 4.2733) (-32.2346, 4.2915) (-32.2749, 4.3111) (-32.3123, 4.3321) (-32.3467, 4.3548) (-32.3781, 4.379) (-32.4067, 4.4047) (-32.4236, 4.4234) (-32.4319, 4.4326) knots 0 0 0 0 0.144606 0.282107 0.414027 0.540032 0.660947 0.777882 0.890226 1 1 1 1
  spline S56 degree 3 poles (-32.6898, -5.9478) (-32.6895, -5.9578) (-32.6889, -5.9773) (-32.6829, -6.0055) (-32.6734, -6.0321) (-32.6639, -6.0482) (-32.6591, -6.0563) knots 0 0 0 0 0.260773 0.510344 0.754071 1 1 1 1
  spline S57 degree 3 poles (-32.3888, 3.8479) (-32.3886, 3.8401) (-32.3882, 3.8247) (-32.3854, 3.8021) (-32.3805, 3.7803) (-32.374, 3.7593) (-32.3653, 3.7391) (-32.3546, 3.7198) (-32.3422, 3.7011) (-32.328, 3.6837) (-32.3128, 3.6675) (-32.2966, 3.6535) (-32.2798, 3.6416) (-32.2628, 3.6315) (-32.2448, 3.6242) (-32.2264, 3.6188) (-32.2075, 3.6151) (-32.1946, 3.6148) (-32.1881, 3.6147) knots 0 0 0 0 0.06843 0.135537 0.200741 0.265609 0.329763 0.394392 0.460266 0.526906 0.592772 0.655867 0.715884 0.773708 0.830514 0.886457 0.942756 1 1 1 1
  spline S58 degree 3 poles (-32.0705, 2.8623) (-32.079, 2.8717) (-32.0951, 2.8897) (-32.1163, 2.9168) (-32.134, 2.942) (-32.1477, 2.9661) (-32.1583, 2.9895) (-32.1654, 3.013) (-32.1702, 3.0367) (-32.1707, 3.0526) (-32.1709, 3.0606) knots 0 0 0 0 0.167067 0.318047 0.452732 0.572091 0.682749 0.790426 0.895144 1 1 1 1
  spline S59 degree 3 poles (-32.4325, 2.9268) (-32.4383, 2.934) (-32.4496, 2.9484) (-32.4642, 2.9713) (-32.4765, 2.9949) (-32.4868, 3.0191) (-32.4946, 3.0441) (-32.5003, 3.0697) (-32.5034, 3.096) (-32.504, 3.1137) (-32.5042, 3.1227) knots 0 0 0 0 0.130181 0.257507 0.381613 0.505119 0.627383 0.749705 0.873836 1 1 1 1
  spline S60 degree 3 poles (-31.9145, 3.781) (-31.9143, 3.7725) (-31.9139, 3.756) (-31.9121, 3.732) (-31.9081, 3.7096) (-31.9034, 3.6884) (-31.8966, 3.669) (-31.8889, 3.6509) (-31.8792, 3.6346) (-31.8684, 3.6196) (-31.8564, 3.6065) (-31.8438, 3.5949) (-31.8304, 3.5853) (-31.8166, 3.5771) (-31.8017, 3.5711) (-31.7863, 3.5668) (-31.7703, 3.5637) (-31.7594, 3.5635) (-31.7538, 3.5634) knots 0 0 0 0 0.084029 0.163004 0.23813 0.30951 0.377269 0.44153 0.504366 0.564948 0.623935 0.680121 0.73409 0.786835 0.839029 0.891988 0.945047 1 1 1 1
  spline S61 degree 3 poles (-31.9774, 3.6149) (-31.9832, 3.6056) (-31.9946, 3.5877) (-32.015, 3.5641) (-32.0368, 3.5438) (-32.0607, 3.5274) (-32.0864, 3.5146) (-32.1139, 3.5059) (-32.1431, 3.5002) (-32.1632, 3.4996) (-32.1735, 3.4993) knots 0 0 0 0 0.13704 0.265937 0.389817 0.50968 0.628405 0.748113 0.87081 1 1 1 1
  spline S62 degree 3 poles (-32.5042, 4.6289) (-32.5039, 4.6381) (-32.5034, 4.6563) (-32.4994, 4.6831) (-32.4922, 4.7086) (-32.4829, 4.7332) (-32.4702, 4.7565) (-32.4552, 4.7789) (-32.4372, 4.8) (-32.4166, 4.8197) (-32.3937, 4.8381) (-32.3677, 4.8537) (-32.3395, 4.8672) (-32.3087, 4.8779) (-32.2755, 4.8866) (-32.2398, 4.8924) (-32.2016, 4.8961) (-32.1754, 4.8965) (-32.1619, 4.8967) knots 0 0 0 0 0.056673 0.111837 0.165868 0.219108 0.273055 0.328 0.384454 0.44305 0.503198 0.564677 0.628705 0.694865 0.7648 0.838836 0.917113 1 1 1 1
  line L126 (-32.3628, -6.2372) -> (-32.1898, -6.2757)
  line L127 (-32.1898, -6.8526) -> (-32.3628, -6.8141)
  spline S63 degree 3 poles (-32.3277, 2.9887) (-32.32, 2.9817) (-32.3041, 2.9674) (-32.278, 2.948) (-32.2494, 2.9303) (-32.2185, 2.9135) (-32.1849, 2.8986) (-32.149, 2.8851) (-32.1107, 2.8725) (-32.0841, 2.8657) (-32.0705, 2.8623) knots 0 0 0 0 0.108261 0.220373 0.336206 0.457125 0.58366 0.71601 0.854809 1 1 1 1
  spline S64 degree 3 poles (-32.4319, 4.4326) (-32.4377, 4.4398) (-32.4493, 4.4539) (-32.4637, 4.4769) (-32.4764, 4.5003) (-32.4866, 4.5245) (-32.4944, 4.5496) (-32.5, 4.5754) (-32.5035, 4.6019) (-32.504, 4.6198) (-32.5042, 4.6289) knots 0 0 0 0 0.129587 0.256497 0.379807 0.502911 0.624776 0.748531 0.872375 1 1 1 1
  spline S65 degree 3 poles (-32.8094, -6.026) (-32.8138, -6.0044) (-32.8225, -5.9623) (-32.8238, -5.9193) (-32.8244, -5.8983) knots 0 0 0 0 0.511633 1 1 1 1
  spline S66 degree 3 poles (-32.6552, -5.6915) (-32.6517, -5.6916) (-32.6437, -5.6917) (-32.6301, -5.6931) (-32.6136, -5.6952) (-32.5941, -5.6983) (-32.5715, -5.7018) (-32.5461, -5.7064) (-32.5177, -5.7118) (-32.4978, -5.7159) (-32.4872, -5.718) knots 0 0 0 0 0.061813 0.141568 0.239446 0.355545 0.489631 0.642006 0.810966 1 1 1 1
  line L128 (-32.4872, -5.718) -> (-31.8436, -5.8526)
  line L129 (-31.4359, -5.9436) -> (-31.3051, -6.1411)
  line L130 (-31.3051, -6.1411) -> (-31.709, -6.0641)
  spline S67 degree 3 poles (-32.1619, 4.8967) (-32.1408, 4.8962) (-32.0984, 4.8953) (-32.0345, 4.888) (-31.9702, 4.8759) (-31.9168, 4.8621) (-31.8749, 4.8493) (-31.8448, 4.8396) (-31.8164, 4.8294) (-31.7896, 4.8188) (-31.7644, 4.8084) (-31.7409, 4.7972) (-31.7189, 4.7862) (-31.6924, 4.7711) (-31.6623, 4.7518) (-31.6295, 4.7282) (-31.6012, 4.7036) (-31.5767, 4.679) (-31.5563, 4.6538) (-31.5385, 4.6293) (-31.5238, 4.6047) (-31.5117, 4.5802) (-31.5025, 4.5552) (-31.4962, 4.5289) (-31.492, 4.5014) (-31.4916, 4.4826) (-31.4914, 4.4731) knots 0 0 0 0 0.072797 0.146678 0.222091 0.299106 0.337241 0.373682 0.408526 0.441504 0.473071 0.502927 0.531432 0.558214 0.608374 0.654981 0.698039 0.737885 0.774964 0.80989 0.842722 0.87381 0.904056 0.934974 0.966947 1 1 1 1
  spline S68 degree 3 poles (-31.4914, 4.4731) (-31.4917, 4.4637) (-31.4923, 4.4452) (-31.4961, 4.4181) (-31.5027, 4.3922) (-31.5122, 4.3676) (-31.5241, 4.3441) (-31.5386, 4.3217) (-31.556, 4.3007) (-31.5758, 4.2809) (-31.598, 4.2627) (-31.6228, 4.2471) (-31.65, 4.2338) (-31.6796, 4.2231) (-31.7115, 4.2146) (-31.7456, 4.2087) (-31.7821, 4.2051) (-31.8072, 4.2046) (-31.8201, 4.2044) knots 0 0 0 0 0.058747 0.115884 0.171283 0.226467 0.28101 0.336459 0.393341 0.452019 0.511909 0.572949 0.635928 0.701561 0.770078 0.842426 0.919075 1 1 1 1
  spline S69 degree 3 poles (-32.8244, -5.8983) (-32.8239, -5.8823) (-32.8229, -5.8516) (-32.812, -5.8084) (-32.7952, -5.7697) (-32.7777, -5.7488) (-32.7691, -5.7384) knots 0 0 0 0 0.276555 0.530327 0.767135 1 1 1 1
  line L131 (-31.709, -6.0641) -> (-31.709, -6.2564)
  spline S70 degree 3 poles (-31.8398, 2.7044) (-31.8533, 2.7046) (-31.8802, 2.7049) (-31.9205, 2.7073) (-31.9607, 2.7116) (-32.0007, 2.7174) (-32.0406, 2.7248) (-32.0803, 2.7339) (-32.12, 2.7443) (-32.1462, 2.7528) (-32.1593, 2.7571) knots 0 0 0 0 0.124443 0.248467 0.372332 0.496807 0.621479 0.746544 0.872793 1 1 1 1
  spline S71 degree 3 poles (-32.1881, 3.6147) (-32.1825, 3.6149) (-32.1715, 3.6152) (-32.1553, 3.6173) (-32.1399, 3.6214) (-32.1253, 3.6269) (-32.1114, 3.6337) (-32.0981, 3.6421) (-32.0858, 3.6523) (-32.0743, 3.6638) (-32.0639, 3.6767) (-32.0546, 3.6907) (-32.047, 3.7058) (-32.0408, 3.722) (-32.0357, 3.7391) (-32.0325, 3.7574) (-32.0301, 3.7766) (-32.0299, 3.7898) (-32.0299, 3.7966) knots 0 0 0 0 0.062187 0.121902 0.180732 0.237596 0.294478 0.352328 0.410654 0.47131 0.532289 0.59423 0.656403 0.719848 0.785367 0.853824 0.925279 1 1 1 1
  line L132 (-17.2426, -5.6495) -> (-17.2426, -5.7841)
  line L133 (-17.8782, -4.4827) -> (-17.2426, -4.6242)
  line L134 (-17.5119, -6.8225) -> (-17.5119, -7.2264)
  spline S72 degree 3 poles (-17.9563, -4.6453) (-17.9704, -4.6424) (-17.9969, -4.637) (-18.0341, -4.6305) (-18.0663, -4.6266) (-18.0861, -4.626) (-18.0951, -4.6257) knots 0 0 0 0 0.307639 0.576784 0.807205 1 1 1 1
  line L135 (-17.5119, -6.2456) -> (-17.5119, -6.6495)
  spline S73 degree 3 poles (-32.3911, -5.2354) (-32.3859, -5.2374) (-32.3746, -5.2417) (-32.356, -5.247) (-32.3351, -5.2537) (-32.311, -5.2593) (-32.2846, -5.2661) (-32.2552, -5.2726) (-32.2232, -5.2795) (-32.201, -5.2841) (-32.1895, -5.2865) knots 0 0 0 0 0.079906 0.173499 0.27898 0.3966 0.528922 0.672479 0.830442 1 1 1 1
  line L136 (-18.0888, -6.6495) -> (-17.685, -6.6495)
  line L137 (-17.108, -6.8225) -> (-17.5119, -6.8225)
  line L138 (-17.3773, -5.611) -> (-17.2426, -5.6495)
  spline S74 degree 3 poles (-32.5615, -4.7327) (-32.571, -4.7332) (-32.5893, -4.7342) (-32.6154, -4.7404) (-32.6376, -4.7528) (-32.6568, -4.7688) (-32.6716, -4.7899) (-32.6825, -4.815) (-32.6887, -4.8445) (-32.6894, -4.8655) (-32.6898, -4.8766) knots 0 0 0 0 0.130697 0.251063 0.363318 0.475137 0.590039 0.712809 0.847528 1 1 1 1
  line L139 (-31.709, -4.7312) -> (-31.709, -4.9073)
  line L140 (-31.709, -5.385) -> (-31.709, -5.5611)
  line L141 (-16.9695, -5.8367) -> (-16.8388, -6.0341)
  spline S75 degree 3 poles (-18.0083, -5.7841) (-18.0178, -5.7823) (-18.0358, -5.779) (-18.0614, -5.7749) (-18.084, -5.7713) (-18.1035, -5.7683) (-18.12, -5.7659) (-18.1334, -5.764) (-18.144, -5.763) (-18.15, -5.7628) (-18.1525, -5.7627) knots 0 0 0 0 0.198784 0.376221 0.532667 0.670161 0.782601 0.87611 0.948465 1 1 1 1
  line L142 (-32.3445, -4.5897) -> (-31.709, -4.7312)
  line L143 (-17.685, -6.2456) -> (-17.5119, -6.2456)
  line L144 (-18.3388, -5.0533) -> (-18.1405, -5.0939)
  spline S76 degree 3 poles (-32.8244, -3.8114) (-32.8238, -3.791) (-32.8226, -3.7506) (-32.8121, -3.6917) (-32.7949, -3.6356) (-32.7712, -3.5828) (-32.7417, -3.5343) (-32.706, -3.4914) (-32.6642, -3.4549) (-32.6171, -3.425) (-32.5654, -3.4011) (-32.5097, -3.384) (-32.45, -3.3735) (-32.4089, -3.3724) (-32.3878, -3.3718) knots 0 0 0 0 0.08805 0.173362 0.256795 0.339941 0.4214 0.500643 0.579137 0.659 0.740185 0.823206 0.909367 1 1 1 1
  spline S77 degree 3 poles (-18.343, -5.919) (-18.3475, -5.8974) (-18.3562, -5.8553) (-18.3574, -5.8123) (-18.358, -5.7913) knots 0 0 0 0 0.511633 1 1 1 1
  spline S78 degree 3 poles (-18.1525, -5.7627) (-18.1579, -5.763) (-18.1682, -5.7634) (-18.1826, -5.7667) (-18.195, -5.7722) (-18.2056, -5.7801) (-18.214, -5.7911) (-18.2196, -5.8051) (-18.2228, -5.822) (-18.2232, -5.8342) (-18.2234, -5.8409) knots 0 0 0 0 0.133915 0.253294 0.361774 0.467629 0.576952 0.697757 0.836473 1 1 1 1